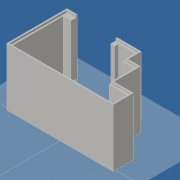
# Autodesk Inventor part: Display
Saved by Autodesk Inventor 2016 SP2 (Build 200236200, 236)
## iProperties
Created: 2018-07-08
Part Number: Display
Material: Generisch
Document SubType Name: Modeling
Designer: User
Density: 1 g/cm^3
Appearance: Vorgabe
Author: User
Autodesk Inventor part; units mm, degrees
ref_plane "YZ Plane" through (0, 0, 0) normal (1, 0, 0) x (0, 1, 0)
ref_plane "XZ Plane" through (0, 0, 0) normal (0, 1, 0) x (-1, 0, 0)
ref_plane "XY Plane" through (0, 0, 0) normal (0, 0, 1) x (1, 0, 0)
sketch "Skizze1" plane through (0, 0, 0) normal (0, 0, 1) x (1, 0, 0)
  line L0 (-65, 0) -> (65, 0)
  line L1 (65, 0) -> (65, 20)
  line L2 (65, 20) -> (40, 20)
  line L3 (40, 20) -> (40, 54)
  line L4 (-65, 41) -> (-65, 0)
  line L5 (-65, 41) -> (-65, 41)
  line L6 (-65, 54) -> (-65, 54)
  line L7 (-65, 54) -> (-65, 41)
  line L8 (24, 71) -> (24, 54)
  line L9 (24, 54) -> (40, 54)
  circle A0 centre (-59.5, 2.832) radius 1.25
  circle A1 centre (23.1262, 2.832) radius 1.25
  circle A2 centre (23.1262, 51.168) radius 1.25
  circle A3 centre (-52.007, 51.168) radius 1.25
  line L10 (25.8762, 2.832) -> (25.8762, 0)
  line L11 (25.8762, 0) -> (20.3762, 0)
  line L12 (20.3762, 0) -> (20.3762, 2.832)
  arc A4 (25.8762, 2.832) -> (20.3762, 2.832) centre (23.1262, 2.832) ccw
  line L13 (-56.75, 0) -> (-56.75, 2.832)
  line L14 (-62.25, 0) -> (-62.25, 2.832)
  line L15 (-56.75, 0) -> (-62.25, 0)
  arc A5 (-56.75, 2.832) -> (-62.25, 2.832) centre (-59.5, 2.832) ccw
  line L16 (25.8762, 51.168) -> (25.8762, 54)
  line L17 (25.8762, 54) -> (20.3762, 54)
  line L18 (20.3762, 54) -> (20.3762, 51.168)
  arc A6 (20.3762, 51.168) -> (25.8762, 51.168) centre (23.1262, 51.168) ccw
  line L19 (-49.257, 51.168) -> (-49.257, 54)
  line L20 (-49.257, 54) -> (-54.757, 54)
  line L21 (-54.757, 54) -> (-54.757, 51.168)
  arc A7 (-54.757, 51.168) -> (-49.257, 51.168) centre (-52.007, 51.168) ccw
  line L22 (-65, 54) -> (24, 54)
  line L23 (24, 54) -> (24, 57)
  line L24 (24, 57) -> (-65, 57)
  line L25 (-65, 57) -> (-65, 54)
  line L26 (24, 71) -> (-65, 71)
  line L27 (-65, 71) -> (-65, 54)
  line L28 (43, 23) -> (68, 23)
  line L29 (68, 23) -> (68, -3)
  line L30 (68, -3) -> (-68, -3)
  line L31 (-68, -3) -> (-68, 44)
  line L32 (-68, 44) -> (-68, 44)
  line L33 (-68, 44) -> (-68, 57)
  line L34 (-68, 57) -> (-68, 57)
  line L35 (-68, 57) -> (-68, 74)
  line L36 (-68, 74) -> (27, 74)
  line L37 (27, 74) -> (27, 57)
  line L38 (27, 57) -> (43, 57)
  line L39 (43, 57) -> (43, 23)
  line L40 (-65, 71) -> (-55, 71)
  line L41 (-55, 71) -> (-55, 66)
  line L42 (-55, 66) -> (-65, 66)
  line L43 (-65, 66) -> (-65, 71)
  line L44 (1, 71) -> (-4, 71)
  line L45 (-4, 71) -> (-4, 66)
  line L46 (-4, 66) -> (1, 66)
  line L47 (1, 66) -> (1, 71)
  line L48 (-55, 71) -> (-4, 71)
  line L49 (-4, 71) -> (-4, 74)
  line L50 (-4, 74) -> (-55, 74)
  line L51 (-55, 74) -> (-55, 71)
  point P0 (0, 0)
  point P1 (0, 0)
  point P2 (0, 0)
  point P3 (0, 0)
  dimension "d0" = 130
  dimension "d1" = 25
  dimension "d2" = 20
  dimension "d3" = 41
  dimension "d4" = 54
  dimension "d5" = 5.5
  dimension "d6" = 82.6262
  dimension "d7" = 2.5
  dimension "d8" = 2.832
  dimension "d9" = 7.493
  dimension "d10" = 48.336
  dimension "d11" = 5.5
  dimension "d12" = 5.5
  dimension "d13" = 5.5
  dimension "d14" = 5.5
  dimension "d15" = 3
  dimension "d16" = 0
  dimension "d17" = 89
  dimension "d18" = 71
  dimension "d19" = 3
  dimension "d20" = 2.832
  dimension "d29" = 10
  dimension "d30" = 5
  dimension "d31" = 5
  dimension "d34" = 51
  dimension "d40" = 0
  constraints: 105 end point, 19 perpendicular, 9 horizontal, 8 centre point, 8 parallel, 8 point on circle, 8 point on line, 8 tangent, 7 coincident, 6 vertical, 5 collinear, 3 equal radius, 3 horizontal alignment, 1 midpoint, 1 vertical alignment, 11 other
  measures "d0" distance between parallel lines of L1 L4
  measures "d1" distance between parallel lines of L1 L3
  measures "d2" distance between parallel lines of L0 L2
  measures "d3" distance between parallel lines of L0 L5
  measures "d4" distance between parallel lines of L0 L6
  measures "d5" distance from line of L4 A0.centre
  measures "d6" distance of A0.centre A1.centre
  measures "d7" diameter of A0
  measures "d8" distance from line of L0 A0.centre
  measures "d9" horizontal distance of A0.centre A3.centre
  measures "d10" vertical distance of A0.centre A3.centre
  measures "d11" distance between parallel lines of L12 L10
  measures "d12" distance between parallel lines of L14 L13
  measures "d13" distance between parallel lines of L18 L16
  measures "d14" distance between parallel lines of L21 L19
  measures "d15" distance between parallel lines of L22 L24
  measures "d16" distance between parallel lines of L7 L4
  measures "d17" distance of L8.start L26.end
  measures "d18" distance between parallel lines of L0 L26
  measures "d19" distance between parallel lines of L2 L28
  measures "d20" distance from line of L22 A2.centre
  measures "d29" distance of L41.end L42.end
  measures "d30" distance of L45.end L46.end
  measures "d31" distance of L40.end L41.end
  measures "d34" distance between parallel lines of L45 L41
  measures "d40" distance between parallel lines of L35 L33
extrude "Extrusion1" add sketch "Skizze1" along normal blind 68 contours L0 L1 L2 L3 L9 L8 L26 L49 L36 L37 L38 L39 L28 L29 L30 L31 L33 L35 L51 L27 L25 L7 L4 | L27 L26 L41 L42 | L47 L46 L45 L26
sketch "Skizze3" plane through (-4, 74, 0) normal (0, 1, 0) x (1, 0, 0)
  line L0 (31, 0) -> (31, -68) projected
  line L1 (28, 0) -> (5, 0) projected
  arc A0 (13, 0) -> (24.5, 0) centre (18.75, -1.7139) ccw
  line L2 (13, 0) -> (24.5, 0)
  point P0 (4, 0)
  dimension "d35" = 6
  dimension "d36" = 12.25
  dimension "d39" = 11.5
  constraints: 2 end point, 2 point on circle, 2 point on line, 1 centre point, 1 collinear
  measures "d35" radius of A0
  measures "d36" distance from line of L0 A0.centre
  measures "d39" distance of L2.end L2.start
extrude "Extrusion4" cut sketch "Skizze3" against normal up to surface (3 mm away)
sketch "Skizze4" plane through (0, 0, 68) normal (0, 0, 1) x (1, 0, 0)
  line L0 (65, 0) -> (-65, 0) projected
  line L1 (-55, 74) -> (-68, 74) projected
  line L2 (-68, 74) -> (-68, -3) projected
  line L3 (43, 23) -> (43, 57) projected
  line L4 (43, 57) -> (27, 57) projected
  line L5 (27, 74) -> (-4, 74) projected
  line L6 (-55, 74) -> (-68, 74)
  line L7 (-68, 74) -> (-68, -3)
  line L8 (-68, -3) -> (68, -3)
  line L9 (68, -3) -> (68, 23)
  line L10 (68, 23) -> (43, 23)
  line L11 (43, 23) -> (43, 57)
  line L12 (43, 57) -> (27, 57)
  line L13 (27, 57) -> (27, 74)
  line L14 (27, 74) -> (-4, 74)
  line L15 (-4, 72.5) -> (25.5, 72.5)
  line L16 (25.5, 72.5) -> (25.5, 55.5)
  line L17 (25.5, 55.5) -> (41.5, 55.5)
  line L18 (41.5, 55.5) -> (41.5, 21.5)
  line L19 (41.5, 21.5) -> (66.5, 21.5)
  line L20 (66.5, 21.5) -> (66.5, -1.5)
  line L21 (66.5, -1.5) -> (-66.5, -1.5)
  line L22 (-66.5, -1.5) -> (-66.5, 72.5)
  line L23 (-66.5, 72.5) -> (-55, 72.5)
  line L24 (-4, 72.5) -> (-4, 74)
  line L25 (-55, 72.5) -> (-55, 74)
  point P0 (0, 0)
  dimension "d41" = 1.5
  constraints: 40 end point, 6 perpendicular, 5 collinear, 2 parallel, 1 vertical, 8 other
  measures "d41" distance between parallel lines of L14 L15
extrude "Extrusion5" add sketch "Skizze4" along normal blind 3
sketch "Skizze5" plane through (0, 0, 0) normal (0, 0, -1) x (-1, 0, 0)
  line L0 (-27, 74) -> (-27, 57) projected
  line L1 (-43, 23) -> (-68, 23) projected
  line L2 (55, 74) -> (55, 66) projected
  line L3 (-20.5, 74) -> (-27, 74)
  line L4 (-27, 74) -> (-27, 57)
  line L5 (-27, 57) -> (-43, 57)
  line L6 (-43, 57) -> (-43, 23)
  line L7 (-43, 23) -> (-68, 23)
  line L8 (-68, 23) -> (-68, -3)
  line L9 (68, 74) -> (68, -3) projected
  line L10 (-68, -3) -> (68, -3)
  line L11 (68, -3) -> (68, 74)
  line L12 (68, 74) -> (55, 74)
  line L13 (-20.5, 72.5) -> (-25.5, 72.5)
  line L14 (-25.5, 72.5) -> (-25.5, 55.5)
  line L15 (-25.5, 55.5) -> (-41.5, 55.5)
  line L16 (-41.5, 55.5) -> (-41.5, 21.5)
  line L17 (-41.5, 21.5) -> (-66.5, 21.5)
  line L18 (-66.5, 21.5) -> (-66.5, -1.5)
  line L19 (-66.5, -1.5) -> (66.5, -1.5)
  line L20 (66.5, -1.5) -> (66.5, 72.5)
  line L21 (66.5, 72.5) -> (55, 72.5)
  line L22 (-20.5, 74) -> (-20.5, 72.5)
  line L23 (55, 74) -> (68, 74) projected
  line L24 (55, 66) -> (55, 72.5) projected
  line L25 (55, 74) -> (55, 72.5)
  line L26 (4, 74) -> (-9, 74) projected
  line L27 (4, 72.5) -> (4, 66) projected
  line L28 (-9, 74) -> (4, 74)
  line L29 (4, 74) -> (4, 72.5)
  line L30 (4, 72.5) -> (-9, 72.5)
  line L31 (-9, 72.5) -> (-9, 74)
  point P0 (0, 0)
  dimension "d44" = 1.5
  dimension "d47" = 1.5
  constraints: 48 end point, 11 perpendicular, 4 equal length, 2 horizontal, 2 vertical, 1 point on line, 8 other
  measures "d44" distance between parallel lines of L3 L13
  measures "d47" distance between parallel lines of L30 L26
extrude "Extrusion6" add sketch "Skizze5" along normal blind 3
equation "\"d47\" = d44"
